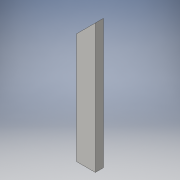
# Autodesk Inventor part: Front Face Bottom Support for Slats
Saved by Autodesk Inventor 2016 (Build 200138000, 138)
## iProperties
Created: 2015-07-06
Part Number: Front Face Bottom Support for Slats
Material: Generic
Document SubType Name: Modeling
Designer: steele
Density: 1 g/cm^3
Appearance: Default
Author: steele
Autodesk Inventor part; units mm, degrees
ref_plane "YZ Plane" through (0, 0, 0) normal (1, 0, 0) x (0, 1, 0)
ref_plane "XZ Plane" through (0, 0, 0) normal (0, 1, 0) x (-1, 0, 0)
ref_plane "XY Plane" through (0, 0, 0) normal (0, 0, 1) x (1, 0, 0)
sketch "Sketch1" plane through (0, 0, 0) normal (0, 0, 1) x (1, 0, 0)
  line L0 (-50.0735, -347.1667) -> (38.8265, -347.1667)
  line L1 (38.8265, -347.1667) -> (38.8265, 269.1897)
  line L2 (-50.0735, 180.2897) -> (-50.0735, -347.1667)
  line L3 (-50.0735, -347.1667) -> (38.8265, 269.1897) construction
  line L4 (38.8265, -347.1667) -> (26.0247, -232.6993) construction
  line L5 (38.8265, 269.1897) -> (-50.0735, 180.2897)
  line L6 (38.8265, 269.1897) -> (164.5501, 269.1897) construction
  point P0 (0, 0)
  dimension "d1" = 88.9
  dimension "d2" = 616.3564
  dimension "d5" = 45
  constraints: 14 end point, 2 horizontal, 2 point on line, 1 equal length, 1 parallel, 1 perpendicular
  measures "d1" distance of L0.start L0.end
  measures "d2" distance of L0.end L1.end
  measures "d5" angle of L1 L5
extrude "Extrusion1" add sketch "Sketch1" along normal mid plane 38.1
body "Solid1"
